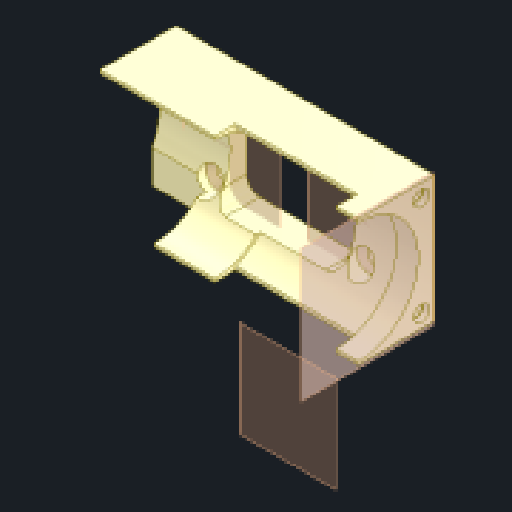
# Autodesk Inventor part: right_motor_mount
Saved by Autodesk Inventor 2023 (Build 270158000, 158)
## iProperties
Created: 2024-04-27
Part Number: right_motor_mount
Material: Nylon 6/6
Document SubType Name: Modeling
Designer: szymo
Density: 1.13 g/cm^3
Appearance: Nylon 6
Mass: 11.8928 g
Surface Area: 74.7703 cm^2
Volume: 10.5246 cm^3
Author: szymo
Autodesk Inventor part; units mm, degrees
ref_plane "YZ Plane" through (0, 0, 0) normal (1, 0, 0) x (0, 1, 0)
ref_plane "XZ Plane" through (0, 0, 0) normal (0, 1, 0) x (-1, 0, 0)
ref_plane "XY Plane" through (0, 0, 0) normal (0, 0, 1) x (1, 0, 0)
ref_plane "Work Plane1" through (-37.7, -67.375, 15.375) normal (1, 0, 0) x (0, 0, 1)
sketch "Sketch1" plane through (-37.7, -67.375, 15.375) normal (1, 0, 0) x (0, 0, 1)
  arc A0 (7.9062, 3.651) -> (9.7035, 4.7619) centre (8.8048, 4.2064) ccw projected
  arc A1 (7.9062, 3.651) -> (4.5768, 6.4477) centre (2, 0) ccw projected
  arc A2 (5.3608, 8.4097) -> (4.5768, 6.4477) centre (4.9688, 7.4287) ccw projected
  arc A3 (9.7035, 4.7619) -> (5.3608, 8.4097) centre (2, 0) ccw projected
  arc A4 (4.5768, -6.4477) -> (5.3608, -8.4097) centre (4.9688, -7.4287) ccw projected
  arc A5 (4.5768, -6.4477) -> (7.9062, -3.651) centre (2, 0) ccw projected
  arc A6 (9.7035, -4.7619) -> (7.9062, -3.651) centre (8.8048, -4.2064) ccw projected
  arc A7 (5.3608, -8.4097) -> (9.7035, -4.7619) centre (2, 0) ccw projected
  arc A8 (-0.5553, 6.4563) -> (-1.3328, 8.4209) centre (-0.9441, 7.4386) ccw projected
  arc A9 (-0.5553, 6.4563) -> (-3.9062, 3.651) centre (2, 0) ccw projected
  arc A10 (-5.7035, 4.7619) -> (-3.9062, 3.651) centre (-4.8048, 4.2064) ccw projected
  arc A11 (-1.3328, 8.4209) -> (-5.7035, 4.7619) centre (2, 0) ccw projected
  arc A12 (-3.9062, -3.651) -> (-5.7035, -4.7619) centre (-4.8048, -4.2064) ccw projected
  arc A13 (-3.9062, -3.651) -> (-0.5553, -6.4563) centre (2, 0) ccw projected
  arc A14 (-1.3328, -8.4209) -> (-0.5553, -6.4563) centre (-0.9441, -7.4386) ccw projected
  arc A15 (-5.7035, -4.7619) -> (-1.3328, -8.4209) centre (2, 0) ccw projected
  circle A16 centre (2.0124, -10.65) radius 1.15 projected
  circle A17 centre (10, 0) radius 1.0564 projected
  circle A18 centre (-6, 0) radius 1.0564 projected
  circle A19 centre (2, 0) radius 5 projected
  circle A20 centre (2, 0) radius 13.7 projected
  line L0 (-17.375, -14.375) -> (-15.375, -14.375) projected
  line L1 (-15.375, 91.625) -> (-15.375, -14.375) projected
  line L2 (-17.375, 91.625) -> (-15.375, 91.625) projected
  circle A21 centre (2, 0) radius 14.375 projected
  line L3 (-15.375, -14.375) -> (2, -14.375)
  line L4 (2, -14.375) -> (2, 14.375)
  line L5 (2, 14.375) -> (-15.375, 14.375)
  line L6 (-15.375, 14.375) -> (-15.375, -14.375)
  line L7 (2, 14.375) -> (16.375, 14.375)
  line L8 (16.375, 14.375) -> (16.375, -14.375)
  line L9 (16.375, -14.375) -> (2, -14.375)
  line L10 (2, -14.375) -> (2, 14.375)
  line L11 (-17.375, 91.625) -> (-17.375, -14.375) projected
  point P0 (-15.375, -67.375)
  point P1 (2, 13.7)
  point P2 (-15.375, 14.375)
  point P3 (2, -13.7)
  constraints: 16 end point, 4 horizontal, 4 parallel, 2 perpendicular, 1 vertical, 1 vertical alignment, 1 other
ref_plane "Work Plane2" through (-42.7, -81.75, 1) normal (1, 0, 0) x (0, 1, 0)
extrude "Extrusion1" add sketch "Sketch1" against normal up to surface (5 mm away) contours L4 A21 A20 | L3 L1 L5 A21 picked at (-12.0468, 0.5505)
sketch "Sketch2" plane through (-42.7, -67.375, 17.375) normal (-1, 0, 0) x (0, 0, 1)
  circle A0 centre (0, 0) radius 14.375 projected
  line L0 (-17.375, 14.375) -> (-17.375, -14.375) projected
  line L1 (-17.375, -14.375) -> (0, -14.375) projected
  line L2 (0, -14.375) -> (0, -13.7) projected
  arc A1 (0, 13.7) -> (0, -13.7) centre (0, 0) ccw projected
  line L3 (0, 13.7) -> (0, 14.375) projected
  line L4 (0, 14.375) -> (-17.375, 14.375) projected
  line L5 (-17.375, 14.375) -> (0, 14.375) projected
  line L6 (-4.7286, 14.375) -> (-4.7286, 13.575)
  line L7 (0, -14.375) -> (-17.375, -14.375) projected
  line L8 (-4.7286, -14.375) -> (-4.7286, -13.575)
  point P0 (-17.375, 67.375)
  point P1 (0, -14.375)
  point P2 (0, 14.375)
  point P3 (-4.7286, -14.375)
  point P4 (-4.7286, 14.375)
  dimension "d4" = 0.8
  dimension "d5" = 0.8
  constraints: 4 end point, 2 perpendicular, 2 point on circle, 2 point on line
  measures "d4" distance of L6.start L6.end
  measures "d5" distance of L8.start L8.end
ref_plane "Work Plane3" through (-70.4, -81.75, 1) normal (-1, 0, 0) x (0, 0, 1)
extrude "Extrusion2" add sketch "Sketch2" along normal up to surface (27.7 mm away) contours A0 L8 L1 L0 L4 L6
sketch "Sketch4" plane through (-70.4, -67.375, 17.375) normal (-1, 0, 0) x (0, 0, 1)
  line L0 (-17.375, -14.375) -> (-17.375, 14.375) projected
  line L1 (-4.7286, -14.375) -> (-17.375, -14.375) projected
  arc A0 (-4.7286, 13.575) -> (-4.7286, -13.575) centre (0, 0) ccw projected
  line L2 (-17.375, 14.375) -> (-4.7286, 14.375) projected
  arc A1 (-12.9047, -4.6) -> (12.9047, -4.6) centre (0, 0) ccw projected
  line L3 (12.9047, -4.6) -> (-12.9047, -4.6) projected
  line L4 (12.9047, 4.6) -> (-12.9047, 4.6) projected
  arc A2 (12.9047, 4.6) -> (-12.9047, 4.6) centre (0, 0) ccw projected
  circle A3 centre (0, 0) radius 14.375 projected
  arc A4 (-4.7286, 13.575) -> (-4.7286, -13.575) centre (0, 0) ccw projected
  line L5 (0, -14.375) -> (0, -13.7) projected
  arc A5 (0, 13.7) -> (0, -13.7) centre (0, 0) ccw projected
  line L6 (0, 13.7) -> (0, 14.375) projected
  line L7 (-4.7286, -13.575) -> (-4.7286, -14.375) projected
  line L8 (-4.7286, -14.375) -> (0, -14.375) projected
  line L9 (0, 14.375) -> (-4.7286, 14.375) projected
  line L10 (-4.7286, 14.375) -> (-4.7286, 13.575) projected
  line L11 (-4.7286, -13.575) -> (-4.7286, -14.375) projected
  line L12 (-4.7286, 14.375) -> (-4.7286, 13.575) projected
  point P0 (-17.375, 67.375)
  point P1 (0, -14.375)
  point P2 (0, 14.375)
  point P3 (-4.7286, 14.375)
  point P4 (-4.7286, -14.375)
  point P5 (0, -13.7)
  point P6 (-12.9047, -4.6)
  point P7 (-12.9047, 4.6)
  point P8 (0, 13.7)
ref_plane "Work Plane4" through (-84.2, -81.075, 1.675) normal (-1, 0, 0) x (0, 0, 1)
extrude "Extrusion3" add sketch "Sketch4" along normal up to surface (13.8 mm away) contours L0 L2 L10 A0 L7 L1 | L7 A3 L8 | L9 A3 L10 | A0 A3 L6 A2 A5 A1 L5
sketch "Sketch5" plane through (-84.2, -67.375, 17.375) normal (-1, 0, 0) x (0, 0, 1)
  line L0 (0, 14.375) -> (0, 13.7) projected
  line L1 (-17.375, 14.375) -> (0, 14.375) projected
  line L2 (-17.375, -14.375) -> (-17.375, 14.375) projected
  line L3 (0, -14.375) -> (-17.375, -14.375) projected
  line L4 (0, -13.7) -> (0, -14.375) projected
  arc A0 (0, 13.7) -> (0, -13.7) centre (0, 0) ccw projected
  circle A1 centre (-14.625, -11.625) radius 2.75
  line L5 (-11.875, -14.375) -> (-11.875, -6.8319)
  line L6 (-11.875, -14.375) -> (-4.3319, -14.375) construction
  point P0 (-17.375, 67.375)
  dimension "d8" = 5.5
  dimension "d9" = 2.75
  dimension "d10" = 2.75
  dimension "d11" = 90
  constraints: 4 end point, 1 centre point, 1 horizontal, 1 perpendicular, 1 point on circle, 1 point on line, 1 tangent
  measures "d8" diameter of A1
  measures "d9" distance from line of A1.centre L2
  measures "d10" distance from line of A1.centre L3
  measures "d11" angle of L6 L5
ref_plane "Work Plane5" through (-96.5, -97.7889, 0) normal (1, 0, 0) x (0, 1, 0)
extrude "Extrusion4" add sketch "Sketch5" along normal up to surface (12.3 mm away) contours L0 A0 L5 A1 L2 L1 | A1 L3 L2 | A1 | L5 L3 A1
sketch "Sketch6" plane through (0, 0, 0) normal (0, 0, 1) x (1, 0, 0)
  line L0 (-77.45, -77.225) -> (-55.625, -77.225) projected
  arc A0 (-55.625, -77.225) -> (-52.625, -74.225) centre (-55.625, -74.225) ccw projected
  line L1 (-52.625, -74.225) -> (-52.625, -60.5875) projected
  arc A1 (-52.625, -60.5875) -> (-55.625, -57.5875) centre (-55.625, -60.5875) ccw projected
  line L2 (-55.625, -57.5875) -> (-77.45, -57.5875) projected
  arc A2 (-77.45, -57.5875) -> (-80.45, -60.5875) centre (-77.45, -60.5875) ccw projected
  line L3 (-80.45, -60.5875) -> (-80.45, -74.225) projected
  arc A3 (-80.45, -74.225) -> (-77.45, -77.225) centre (-77.45, -74.225) ccw projected
  point P0 (0, 0)
extrude "Extrusion5" cut sketch "Sketch6" along normal blind 10
sketch "Sketch8" plane through (-96.5, -81.75, 0) normal (-1, 0, 0) x (0, 0, 1)
  circle A0 centre (2.75, 26) radius 2.75
  circle A1 centre (2.75, 2.75) radius 2.75
  line L0 (0, 28.75) -> (0, 0) projected
  line L1 (17.375, 28.75) -> (0, 28.75) projected
  line L2 (0, 0) -> (5.5, 0) projected
  point P0 (0, 81.75)
  dimension "d19" = 5.5
  dimension "d20" = 5.5
  constraints: 4 tangent, 2 centre point
  measures "d19" diameter of A1
  measures "d20" diameter of A0
hole "Hole1" at (-96.5, -55.75, 2.75) at (-96.5, -79, 2.75) direction (1, 0, 0) diameter 4 depth 7.75 counterbore diameter 4.6 counterbore depth 0.75
ref_plane "Work Plane6" through (-37.7, -67.375, 15.375) normal (1, 0, 0) x (0, 0, 1)
ref_plane "Work Plane7" through (-52.625, -67.4105, 3) normal (0, 0.0024694, 0.999997) x (1, 0, 0)
sketch "Sketch17" plane through (-52.625, -67.4105, 3) normal (0, 0.0024694, 0.999997) x (1, 0, 0)
  line L0 (-17.775, -9.8241) -> (-17.775, -13.5633) projected
  line L1 (9.925, -13.5633) -> (-17.775, -13.5633) projected
  line L2 (9.925, 13.5866) -> (9.925, -13.5633) projected
  line L3 (9.925, 13.5866) -> (-17.775, 13.5866) projected
  line L4 (-3.925, 13.5866) -> (-3.925, -13.5633)
  line L5 (9.925, 0.0117) -> (-3.925, -13.5633)
  line L6 (9.925, 0.0117) -> (-3.925, 13.5866)
  line L7 (-3, -9.8241) -> (-17.775, -9.8241) projected
  line L8 (-17.775, 13.5866) -> (-17.775, 9.8135) projected
  line L9 (-17.775, 9.8135) -> (-3, 9.8135) projected
  line L10 (0, 6.8188) -> (0, -6.8188) projected
  point P0 (52.625, 67.4177)
  point P1 (3, 6.7992)
  point P2 (3, -6.7758)
  constraints: 6 end point, 5 midpoint, 2 other
hole "Hole5" at (-49.625, -60.6114, 2.9833) at (-49.625, -74.1863, 3.0168) direction (0, -0.0024694, -0.999997) diameter 3.1 end through all countersink diameter 5.5 countersink angle 90 clearance for "Countersunk Flat Head Screw ISO 2009/7046" size "M2.5" standard "ISO"
sketch "Sketch18" plane through (-52.625, -67.4105, 3) normal (0, 0.0024694, 0.999997) x (1, 0, 0)
  circle A0 centre (3, 6.7992) radius 2.75 projected
  circle A1 centre (3, 6.7992) radius 1.55 projected
  circle A2 centre (3, -6.7758) radius 2.75 projected
  circle A3 centre (3, -6.7758) radius 1.55 projected
  point P0 (52.625, 67.4177)
extrude "Extrusion9" cut sketch "Sketch18" along normal blind 10 contours A0 | A1 | A2 | A3
ref_plane "Work Plane8" through (-80.45, -67.411, 3.675) normal (0, 0.0026299, 0.9999965) x (1, 0, 0)
sketch "Sketch24" plane through (-80.45, -67.411, 3.675) normal (0, 0.0026299, 0.9999965) x (1, 0, 0)
  line L0 (10.05, -13.7) -> (10.05, -9.8249) projected
  line L1 (10.05, 13.7) -> (-16.05, 13.7) projected
  line L2 (-16.05, -6.8006) -> (-16.05, 13.7) projected
  line L3 (-3.75, -6.8006) -> (-16.05, -6.8006) projected
  line L4 (-3.75, -6.8006) -> (-3.75, -13.7) projected
  line L5 (10.05, -13.7) -> (-3.75, -13.7) projected
  line L6 (-3.75, -13.7) -> (-16.05, -13.7)
  line L7 (-16.05, -13.7) -> (-16.05, -6.8006)
  line L8 (-16.05, 14.4206) -> (-16.05, -14.3293) projected
  line L9 (-16.05, 0.0457) -> (10.05, 13.7)
  line L10 (-16.05, 13.7) -> (10.0688, -0.0359)
  line L11 (10.0688, -0.0359) -> (-16.05, -13.7)
  line L12 (10.05, -13.7) -> (-16.0688, 0.0359)
  line L13 (10.05, -9.8249) -> (3, -9.8249) projected
  line L14 (0, -6.8188) -> (0, 6.8188) projected
  line L15 (3, 9.8127) -> (10.05, 9.8127) projected
  line L16 (10.05, 9.8127) -> (10.05, 13.7) projected
  point P0 (80.45, 67.4205)
  point P1 (-2.9906, 6.832)
  point P2 (-3.0094, -6.832)
  constraints: 12 end point, 3 midpoint, 2 collinear, 2 parallel, 1 point on line, 2 other
hole "Hole8" at (-83.4406, -60.579, 3.6571) at (-83.4594, -74.2431, 3.693) direction (0, -0.0026299, -0.9999965) diameter 2.9 end through all countersink diameter 5.5 countersink angle 90 clearance for "Countersunk Flat Head Screw ISO 2009/7046" size "M2.5" standard "ISO"
sketch "Sketch25" plane through (-80.45, -67.411, 3.675) normal (0, 0.0026299, 0.9999965) x (1, 0, 0)
  circle A0 centre (-2.9906, 6.832) radius 2.75 projected
  circle A1 centre (-3.0094, -6.832) radius 2.75 projected
  point P0 (80.45, 67.4205)
extrude "Extrusion11" cut sketch "Sketch25" along normal blind 10
sketch "Sketch26" plane through (-37.7, -67.375, 15.375) normal (1, 0, 0) x (0, 0, -1)
  line L0 (-2, -14.375) -> (15.375, -14.375) projected
  line L1 (15.375, -14.375) -> (15.375, 14.375) projected
  line L2 (15.375, 14.375) -> (-2, 14.375) projected
  arc A0 (-2, -13.7) -> (-2, 13.7) centre (-2, 0) ccw projected
  circle A1 centre (12.375, 11.375) radius 1.45 projected
  circle A2 centre (12.375, -11.375) radius 1.45 projected
  line L3 (-2, 14.375) -> (-2, 13.7) projected
  line L4 (-2, -13.7) -> (-2, -14.375) projected
  point P0 (15.375, 67.375)
  constraints: 2 coincident
hole "Hole9" at (-37.7, -56, 3) at (-37.7, -78.75, 3) direction (-1, 0, 0) diameter 3 depth 3 counterbore diameter 3.5 counterbore depth 1.4
equation "\"d9\" = 0.5 * d8"
equation "\"d10\" = 0.5 * d8"
body "Solid1"
